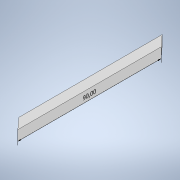
# Autodesk Inventor part: 2ndFloorLongAngle
Saved by Autodesk Inventor 2020.1 (Build 241239000, 239)
## iProperties
Created: 2020-01-31
Part Number: 2ndFloorLongAngle
Material: Generic
Document SubType Name: Modeling
Designer: super
Density: 1 g/cm^3
Appearance: Default
Author: super
Autodesk Inventor part; units mm, degrees
ref_plane "YZ Plane" through (0, 0, 0) normal (1, 0, 0) x (0, 1, 0)
ref_plane "XZ Plane" through (0, 0, 0) normal (0, 1, 0) x (-1, 0, 0)
ref_plane "XY Plane" through (0, 0, 0) normal (0, 0, 1) x (1, 0, 0)
sketch "Sketch1" plane through (0, 0, 0) normal (0, 1, 0) x (-1, 0, 0)
  line L0 (0, 0) -> (0, -90)
  line L1 (0, -90) -> (5.4024, -96)
  line L2 (0, -90) -> (8.0738, -90) construction
  line L3 (5.4024, -96) -> (6.35, -97.0524)
  line L4 (0, 0) -> (6.35, -7.0524)
  line L5 (6.35, -7.0524) -> (6.35, -97.0524)
  dimension "d0" = 90
  constraints: 12 end point, 1 equal length, 1 horizontal, 1 point on line, 1 vertical
  measures "d0" distance of L0.start L0.end
extrude "Extrusion1" add sketch "Sketch1" along normal blind 6.35
body "Solid1"
